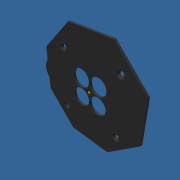
# Autodesk Inventor part: Oktagon_Deckel
Saved by Autodesk Inventor 2018 (Build 220112000, 112)
## iProperties
Created: 2018-10-01
Part Number: Oktagon_Deckel
Material: PC/ABS-Kunststoff
Document SubType Name: Modeling
Designer: N.Grubert
Density: 0.357273 g/cm^3
Appearance: Glatt - weiß
Fläche: 0 cm²
Gewicht: 0 g
Material: geeigneten Werkstoff auswählen !
Dateiname: P:\INVENTOR\Inventor 2018\Templates\ILT\Norm.ipt
Bez_eng: bolt
Bez_french: boulon
Author: N.Grubert
Autodesk Inventor part; units mm, degrees
ref_plane "YZ Plane" through (0, 0, 0) normal (1, 0, 0) x (0, 1, 0)
ref_plane "XZ Plane" through (0, 0, 0) normal (0, 1, 0) x (-1, 0, 0)
ref_plane "XY Plane" through (0, 0, 0) normal (0, 0, 1) x (1, 0, 0)
sketch "Skizze4" plane through (0, 0, 0) normal (0, 1, 0) x (-1, 0, 0)
  line L0 (23.8173, 57.5) -> (57.5, 23.8173)
  line L1 (57.5, 23.8173) -> (57.5, -23.8173)
  line L2 (57.5, -23.8173) -> (23.8173, -57.5)
  line L3 (23.8173, -57.5) -> (-23.8173, -57.5)
  line L4 (-23.8173, -57.5) -> (-57.5, -23.8173)
  line L5 (-57.5, -23.8173) -> (-57.5, 23.8173)
  line L6 (-57.5, 23.8173) -> (-23.8173, 57.5)
  line L7 (-23.8173, 57.5) -> (23.8173, 57.5)
  line L8 (0, -80.5) -> (0, 80.5) construction
  line L9 (80.5, 0) -> (-80.5, 0) construction
  point P0 (0, 0)
  point P1 (0, 0)
  dimension "d4" = 115
  constraints: 16 end point, 1 coincident, 18 other
  measures "d4" distance between parallel lines of L3 L7
extrude "Extrusion2" add sketch "Skizze4" along normal blind 2.5
sketch "Skizze9" plane through (0, 2.5, 0) normal (0, 1, 0) x (1, 0, 0)
  line L0 (-57.5, -23.8173) -> (-23.8173, -57.5) construction
  line L1 (-23.8173, -57.5) -> (23.8173, -57.5) construction
  line L2 (23.8173, -57.5) -> (57.5, -23.8173) construction
  line L3 (57.5, -23.8173) -> (57.5, 23.8173) construction
  line L4 (57.5, 23.8173) -> (23.8173, 57.5) construction
  line L5 (23.8173, 57.5) -> (-23.8173, 57.5) construction
  line L6 (-23.8173, 57.5) -> (-57.5, 23.8173) construction
  line L7 (-57.5, 23.8173) -> (-57.5, -23.8173) construction
  line L8 (-22.5746, -54.5) -> (-54.5, -22.5746)
  line L9 (-54.5, -22.5746) -> (-54.5, 22.5746)
  line L10 (-54.5, 22.5746) -> (-22.5746, 54.5)
  line L11 (-22.5746, 54.5) -> (22.5746, 54.5)
  line L12 (22.5746, 54.5) -> (54.5, 22.5746)
  line L13 (54.5, 22.5746) -> (54.5, -22.5746)
  line L14 (54.5, -22.5746) -> (22.5746, -54.5)
  line L15 (22.5746, -54.5) -> (-22.5746, -54.5)
  line L16 (-51.5, -21.332) -> (-21.332, -51.5)
  line L17 (-21.332, -51.5) -> (21.332, -51.5)
  line L18 (21.332, -51.5) -> (51.5, -21.332)
  line L19 (51.5, -21.332) -> (51.5, 21.332)
  line L20 (51.5, 21.332) -> (21.332, 51.5)
  line L21 (21.332, 51.5) -> (-21.332, 51.5)
  line L22 (-21.332, 51.5) -> (-51.5, 21.332)
  line L23 (-51.5, 21.332) -> (-51.5, -21.332)
  point P0 (0, 0)
  dimension "d20" = 3
  dimension "d21" = 3
  constraints: 32 end point, 14 other
  measures "d20" distance between parallel lines of L0 L8
  measures "d21" distance between parallel lines of L8 L16
extrude "Extrusion6" add sketch "Skizze9" along normal blind 3
sketch "Skizze7" plane through (0, 0, 0) normal (0, -1, 0) x (1, 0, 0)
  line L0 (-23.8173, 57.5) -> (-57.5, 23.8173) construction
  line L1 (-57.5, 23.8173) -> (-57.5, -23.8173) construction
  line L2 (-57.5, -23.8173) -> (-23.8173, -57.5) construction
  line L3 (-23.8173, -57.5) -> (23.8173, -57.5) construction
  line L4 (23.8173, -57.5) -> (57.5, -23.8173) construction
  line L5 (57.5, -23.8173) -> (57.5, 23.8173) construction
  line L6 (57.5, 23.8173) -> (23.8173, 57.5) construction
  line L7 (23.8173, 57.5) -> (-23.8173, 57.5) construction
  line L8 (-57.5, 23.8173) -> (-57.5, -23.8173) projected
  arc A0 (-57.5, 9.798) -> (-57.5, -9.798) centre (-47.5, 0) ccw
  line L9 (-87.767, 0) -> (-49.4975, 0) construction
  line L10 (-80.8477, 9.798) -> (-34.1523, 9.798) construction
  line L11 (-62.7764, -9.798) -> (-50.8218, -9.798) construction
  line L12 (-116.8204, 0) -> (86.5534, 0) construction
  point P0 (0, 0)
  dimension "d15" = 14
  dimension "d16" = 10
  constraints: 6 end point, 4 point on line, 3 horizontal, 3 point on circle, 1 centre point, 1 collinear, 1 midpoint, 1 other
  measures "d15" radius of A0
  measures "d16" distance from line of L1 A0.centre
extrude "Extrusion5" add sketch "Skizze7" against normal up to surface (2.5 mm away)
sketch "Skizze11" plane through (0, 0, 0) normal (0, -1, 0) x (1, 0, 0)
  line L0 (-85.3, 0) -> (81.3, 0) construction
  line L1 (0, -80.5) -> (0, 80.5) construction
  point P0 (0, 0)
  point P1 (-10, 10)
  point P2 (-10, -10)
  point P3 (10, -10)
  point P4 (10, 10)
  dimension "d27" = 10
  dimension "d31" = 10
  dimension "d34" = 360
  constraints: 5 other
  measures "d27" distance from line of L1 point (-10, 10)
  measures "d31" distance from line of point (-10, 10) L0
hole "Bohrung1" at (-10, 0, 10) at (-10, 0, -10) at (10, 0, -10) at (10, 0, 10) direction (0, 1, 0) diameter 19 end through all
sketch "Skizze12" plane through (0, 0, 0) normal (0, -1, 0) x (1, 0, 0)
  line L0 (-23.8173, 57.5) -> (-57.5, 23.8173) projected
  line L1 (57.5, 23.8173) -> (23.8173, 57.5) projected
  line L2 (23.8173, -57.5) -> (57.5, -23.8173) projected
  line L3 (-57.5, -23.8173) -> (-23.8173, -57.5) projected
  line L4 (23.8173, 57.5) -> (23.8173, 23.8173) construction
  line L5 (23.8173, 23.8173) -> (57.5, 23.8173) construction
  line L6 (23.8173, 23.8173) -> (40.6586, 40.6586) construction
  line L7 (23.8173, 57.5) -> (-23.8173, 57.5) construction
  point P0 (0, 0)
  point P1 (32.1734, 32.1734)
  dimension "d44" = 12
  dimension "d47" = 45
  constraints: 7 end point, 2 perpendicular, 1 midpoint, 1 point on line
  measures "d44" distance from line of L1 point (32.173, 32.173)
  measures "d47" angle of L5 L6
hole "Bohrung2" at (32.1734, 0, 32.1734) direction (0, 1, 0) diameter 4 end through all
pattern_circular "Runde Anordnung1" count 4 over 360 about axis through (0, -10, 0) along (0, 1, 0) of "Bohrung2"
chamfer "Fase1" distance 2 angle 45 4 edges at (34.1734, 0, -32.1734) (32.1734, 0, 34.1734) (-34.1734, 0, 32.1734) (-32.1734, 0, -34.1734)
equation "\"d31\" = d27"
equation "\"d44\" = d43"
equation "\"d43\" = 12"
